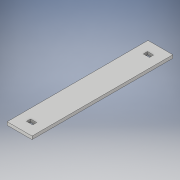
# Autodesk Inventor part: floor_Part
Saved by Autodesk Inventor 2019.4 (Build 234330000, 330)
## iProperties
Created: 2019-12-18
Part Number: floor_Part
Material: Generic
Document SubType Name: Modeling
Designer: fabfarm
Density: 1 g/cm^3
Appearance: Default
Author: fabfarm
Autodesk Inventor part; units mm, degrees
ref_plane "YZ Plane" through (0, 0, 0) normal (1, 0, 0) x (0, 1, 0)
ref_plane "XZ Plane" through (0, 0, 0) normal (0, 1, 0) x (-1, 0, 0)
ref_plane "XY Plane" through (0, 0, 0) normal (0, 0, 1) x (1, 0, 0)
sketch "Sketch1" plane through (0, 0, 0) normal (0, 1, 0) x (-1, 0, 0)
  line L0 (-75, -425) -> (75, -425)
  line L1 (75, -425) -> (75, 425)
  line L2 (75, 425) -> (-75, 425)
  line L3 (-75, 425) -> (-75, -425)
  line L4 (-75, -425) -> (75, 425) construction
  line L5 (75, -425) -> (-75, 425) construction
  point P0 (0, 0)
  dimension "d0" = 850
  dimension "d1" = 150
  constraints: 12 end point, 2 midpoint, 2 parallel, 1 horizontal, 1 perpendicular
  measures "d0" distance of L0.end L1.end
  measures "d1" distance of L0.start L0.end
extrude "Extrusion1" add sketch "Sketch1" along normal blind 18.55
sketch "Sketch2" plane through (0, 18.55, 0) normal (0, 1, 0) x (1, 0, 0)
  line L0 (18.55, -365) -> (-18.55, -365)
  line L1 (-18.55, -365) -> (-18.55, -340)
  line L2 (-18.55, -340) -> (18.55, -340)
  line L3 (18.55, -340) -> (18.55, -365)
  line L4 (18.55, -365) -> (-18.55, -340) construction
  line L5 (-18.55, -365) -> (18.55, -340) construction
  line L6 (18.55, 340) -> (-18.55, 340)
  line L7 (-18.55, 340) -> (-18.55, 365)
  line L8 (-18.55, 365) -> (18.55, 365)
  line L9 (18.55, 365) -> (18.55, 340)
  line L10 (18.55, 340) -> (-18.55, 365) construction
  line L11 (-18.55, 340) -> (18.55, 365) construction
  line L12 (0, -365) -> (0, -425) construction
  line L13 (-75, -425) -> (75, -425) projected
  line L14 (0, 365) -> (0, 425) construction
  line L15 (75, 425) -> (-75, 425) projected
  point P0 (0, 0)
  point P1 (0, -352.5)
  point P2 (0, 352.5)
  dimension "d4" = 730
  dimension "d5" = 25
  dimension "d6" = 37.1
  constraints: 28 end point, 8 midpoint, 4 parallel, 2 collinear, 2 horizontal, 2 perpendicular, 2 vertical, 1 point on line
  measures "d4" distance between parallel lines of L0 L8
  measures "d5" distance of L2.end L0.start
  measures "d6" distance of L1.end L2.end
extrude "Extrusion2" cut sketch "Sketch2" against normal blind 18.55
body "Solid1"
